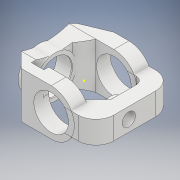
# Autodesk Inventor part: wrist1
Saved by Autodesk Inventor 2017 (Build 210142000, 142)
## iProperties
Created: 2016-12-25
Part Number: wrist1
Material: ABS Plastic
Document SubType Name: Modeling
Designer: Samanth
Density: 1.06 g/cm^3
Appearance: White
Author: Samanth
Autodesk Inventor part; units mm, degrees
ref_plane "YZ Plane" through (0, 0, 0) normal (1, 0, 0) x (0, 1, 0)
ref_plane "XZ Plane" through (0, 0, 0) normal (0, 1, 0) x (-1, 0, 0)
ref_plane "XY Plane" through (0, 0, 0) normal (0, 0, 1) x (1, 0, 0)
sketch "Sketch1" plane through (0, 0, 0) normal (0, 0, 1) x (1, 0, 0)
  line L0 (0, 0) -> (0, 20)
  line L1 (0, 0) -> (0, -12)
  line L2 (0, -12) -> (20, -12)
  line L3 (20, -12) -> (20, 20)
  line L4 (20, 20) -> (0, 20)
  line L5 (0, 20) -> (0, 30)
  line L6 (0, 30) -> (30, 30)
  line L7 (0, -12) -> (0, -22)
  line L8 (0, -22) -> (30, -22)
  line L9 (30, -22) -> (30, 30)
  dimension "d0" = 20
  dimension "d1" = 12
  dimension "d2" = 20
  dimension "d3" = 10
  dimension "d4" = 30
  dimension "d5" = 10
  dimension "d6" = 30
  constraints: 20 end point, 5 perpendicular, 3 vertical, 1 point on line
  measures "d0" distance of L0.start L0.end
  measures "d1" distance of L0.start L1.end
  measures "d2" distance of L1.end L2.end
  measures "d3" distance of L0.end L5.end
  measures "d4" distance of L5.end L6.end
  measures "d5" distance of L1.end L7.end
  measures "d6" distance of L7.end L8.end
extrude "Extrusion1" add sketch "Sketch1" against normal blind 15 contours L5 L6 L9 L8 L7 L2 L3 L4
sketch "Sketch3" plane through (0, 30, 0) normal (0, 1, 0) x (1, 0, 0)
  line L0 (0, 0) -> (0, 15) projected
  circle A0 centre (0, 7.5) radius 11.5
  circle A1 centre (0, 7.5) radius 15.5
  dimension "d14" = 23
  dimension "d15" = 31
  constraints: 2 centre point, 1 coincident, 1 midpoint
  measures "d14" diameter of A0
  measures "d15" diameter of A1
extrude "Extrusion3" add sketch "Sketch3" against normal blind 52 separate body
sketch "Sketch4" plane through (0, 0, 0) normal (0, 0, 1) x (1, 0, 0)
  line L0 (20, -12) -> (20, 20) projected
  line L1 (20, 20) -> (-18.1552, 20)
  line L2 (-18.1552, 20) -> (-18.1552, -12)
  line L3 (-18.1552, -12) -> (20, -12)
  line L4 (20, -12) -> (20, 20)
  point P0 (0, 0)
  constraints: 8 end point, 2 parallel, 1 horizontal, 1 perpendicular
extrude "Extrusion4" cut sketch "Sketch4" along normal mid plane 61.25 bodies 1 2
sketch "Sketch5" plane through (0, -22, -7.5) normal (0, -1, 0) x (1, 0, 0)
  circle A0 centre (0, 0) radius 11.5
  point P0 (0, 7.5)
  constraints: 1 centre point
extrude "Extrusion5" cut sketch "Sketch5" against normal blind 61.25 bodies 2 1
fillet "Fillet1" radius 12 2 edges at (30, -22, -7.5) (30, 30, -7.5)
chamfer "Chamfer1" distance 10 angle 45 1 edges at (20, -12, -7.5)
fillet "Fillet2" radius 5 1 edges at (20, 20, -7.5)
sketch "Sketch7" plane through (30, -10, 0) normal (1, 0, 0) x (0, 0, -1)
  line L0 (0, -12) -> (15, -12) projected
  line L1 (7.5, -12) -> (7.5, 10)
  circle A0 centre (7.5, 10) radius 7.5
  line L2 (0, 0) -> (0, 28) projected
  circle A1 centre (7.5, 10) radius 4.4
  point P0 (0, 10)
  dimension "d27" = 22
  dimension "d28" = 8.8
  constraints: 2 centre point, 2 coincident, 2 end point, 1 midpoint, 1 tangent, 1 vertical
  measures "d27" distance of L1.start L1.end
  measures "d28" diameter of A1
extrude "Extrusion6" add sketch "Sketch7" against normal blind 15 bodies 1
sketch "Sketch8" plane through (15, 0, -7.5) normal (-1, 0, 0) x (0, 0, -1)
  circle A0 centre (0, 0) radius 4.4
  point P0 (-7.5, 0)
  constraints: 1 centre point
extrude "Extrusion7" cut sketch "Sketch8" against normal blind 27.5 bodies 1
sketch "Sketch9" plane through (0, 0, 0) normal (1, 0, 0) x (0, 1, 0)
  point P0 (0, 0)
sketch "Sketch10" plane through (0, 0, 0) normal (0, 0, 1) x (1, 0, 0)
  line L0 (-15.5, 30) -> (15.5, 30) projected
  line L1 (0, 30) -> (-20, 30)
  line L2 (-20, 20) -> (-20, -12)
  line L3 (-20, -12) -> (0, -12)
  line L4 (-15.5, -12) -> (15.5, -12) projected
  line L5 (0, 30) -> (0, 20)
  line L6 (-15.5, -22) -> (15.5, -22) projected
  line L7 (0, -22) -> (-30, -22)
  line L8 (-30, -22) -> (-30, 30)
  line L9 (-30, 30) -> (-20, 30)
  line L10 (15.5, 20) -> (-15.5, 20) projected
  line L11 (-15.5, 20) -> (-20, 20)
  line L12 (-11.5, 20) -> (11.5, 20) projected
  line L13 (0, 20) -> (0, 30)
  line L14 (0, -12) -> (0, -22)
  line L15 (-15, -22) -> (0, -22)
  line L16 (0, -12) -> (0, -22)
  point P0 (0, 0)
  dimension "d40" = 20
  dimension "d41" = 30
  constraints: 24 end point, 6 midpoint, 5 perpendicular, 4 collinear, 2 vertical
  measures "d40" distance of L1.start L1.end
  measures "d41" distance of L7.start L7.end
extrude "Extrusion8" add sketch "Sketch10" along normal blind 8 and the other way blind 22.875 bodies 2
sketch "Sketch11" plane through (30, -10, 0) normal (1, 0, 0) x (0, 0, -1)
  circle A0 centre (7.5, 10) radius 4.4 projected
  circle A1 centre (7.5, 10) radius 4.4
  point P0 (0, 10)
  constraints: 1 centre point, 1 coincident
extrude "Extrusion9" cut sketch "Sketch11" against normal blind 146.75 bodies 1 2
sketch "Sketch12" plane through (0, 30, -7.5) normal (0, 1, 0) x (1, 0, 0)
  line L0 (0, 11.5) -> (0, -11.5) projected
  circle A0 centre (0, 0) radius 11.5946
  point P0 (0, -7.5)
  constraints: 1 centre point, 1 midpoint
extrude "Extrusion10" cut sketch "Sketch12" against normal blind 146.75 bodies 1 2
chamfer "Chamfer4" distance 3 angle 45 1 edges at (15, 7.5, -7.5)
chamfer "Chamfer5" distance 10 angle 45 2 edges at (-30, -22, -7.4375) (-30, 30, -7.4375)
sketch "Sketch13" plane through (0, 0, 8) normal (0, 0, 1) x (1, 0, 0)
  line L0 (0, -12) -> (-20, -12) projected
  line L1 (-11.5946, -12) -> (-11.5946, -22) projected
  line L2 (-20, -12) -> (-11.5946, -12)
  line L3 (-11.5946, -12) -> (-11.5946, -15.2711)
  line L4 (-11.5946, -15.2711) -> (-20, -15.2711)
  line L5 (-20, -15.2711) -> (-20, -12)
  point P0 (0, 0)
  constraints: 8 end point, 2 parallel, 1 horizontal, 1 perpendicular, 1 point on line
extrude "Extrusion11" cut sketch "Sketch13" against normal blind 146.75 bodies 2
chamfer "Chamfer6" distance 8 angle 45 1 edges at (-20, 20, -7.4375)
sketch "Sketch14" plane through (-30, -12, -22.875) normal (-1, 0, 0) x (0, 0, 1)
  line L0 (0, 0) -> (15.375, 0) projected
  arc A0 (0, 0) -> (0.0906, 31.991) centre (-55.2681, 16.1522) ccw
  line L1 (0, 32) -> (30.875, 32) projected
  line L2 (30.875, 0) -> (30.875, -10) projected
  arc A1 (30.875, 32) -> (30.875, 0) centre (76.671, 16) ccw
  line L3 (0, 32) -> (0.088, 32)
  line L4 (22.875, 32) -> (7.875, 32) projected
  line L5 (0, 32) -> (0, 0)
  line L6 (30.875, 0) -> (30.875, 32)
  line L7 (0, 0) -> (0, 32) projected
  line L8 (0, 32) -> (0, 0)
  point P0 (22.875, 12)
  constraints: 8 end point, 5 point on circle, 2 centre point, 2 collinear, 1 parallel
extrude "Extrusion12" cut sketch "Sketch14" against normal blind 146.75 bodies 2
sketch "Sketch15" plane through (-30, -12, -22.875) normal (-1, 0, 0) x (0, 0, 1)
  line L0 (30.875, 0) -> (0, 0) projected
  line L1 (0, 24) -> (0, 32) projected
  arc A0 (0, 0) -> (0, 32) centre (-36.608, 16) ccw
  line L2 (0, 0) -> (0, 32)
  line L3 (0, 24) -> (0, -3.2711) projected
  point P0 (22.875, 12)
  constraints: 2 end point, 2 point on circle, 1 centre point, 1 collinear
extrude "Extrusion13" cut sketch "Sketch15" against normal blind 146.75 bodies 2 1
sketch "Sketch16" plane through (-30, 4, 53.796) normal (-1, 0, 0) x (0, 0, 1)
  circle A0 centre (-61.3202, -4) radius 14
  circle A1 centre (-61.3202, -4) radius 11.5
  point P0 (-53.796, -4)
  dimension "d65" = 28
  dimension "d66" = 23
  constraints: 2 centre point, 1 coincident
  measures "d65" diameter of A0
  measures "d66" diameter of A1
extrude "Extrusion14" add sketch "Sketch16" against normal blind 10.75 separate body
sketch "Sketch17" plane through (-30, 4, 53.796) normal (-1, 0, 0) x (0, 0, 1)
  circle A0 centre (-61.296, -4) radius 4.4 projected
  circle A1 centre (-61.296, -4) radius 11.5
  point P0 (-53.796, -4)
  constraints: 1 centre point, 1 coincident
extrude "Extrusion15" cut sketch "Sketch17" against normal blind 13.25 bodies 2
chamfer "Chamfer7" distance 10 angle 45 1 edges at (-20, 30, -7.4375)
body "Solid1"
body "Solid2"
body "Solid3"
